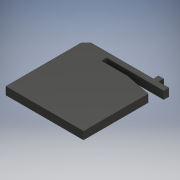
# Autodesk Inventor part: TA11
Saved by Autodesk Inventor 2017 (Build 210142000, 142)
## iProperties
Created: 2019-05-02
Part Number: TA11
Material: ABS Plastic
Document SubType Name: Modeling
Designer: Dell
Density: 1.06 g/cm^3
Appearance: Smooth - Black
Author: Dell
Autodesk Inventor part; units mm, degrees
ref_plane "YZ Plane" through (0, 0, 0) normal (1, 0, 0) x (0, 1, 0)
ref_plane "XZ Plane" through (0, 0, 0) normal (0, 1, 0) x (-1, 0, 0)
ref_plane "XY Plane" through (0, 0, 0) normal (0, 0, 1) x (1, 0, 0)
sketch "Sketch1" plane through (0, 0, 0) normal (0, 0, 1) x (1, 0, 0)
  line L0 (0, 0) -> (30, 0)
  line L1 (30, 0) -> (30, 27)
  line L2 (30, 27) -> (0, 27)
  line L3 (0, 27) -> (0, 0)
  dimension "d0" = 30
  dimension "d1" = 27
  constraints: 8 end point, 2 parallel, 1 horizontal, 1 perpendicular
  measures "d0" distance of L2.end L1.end
  measures "d1" distance of L1.end L0.end
extrude "Extrusion1" add sketch "Sketch1" along normal blind 3
sketch "Sketch2" plane through (0, 27, 0) normal (0, 1, 0) x (1, 0, 0)
  line L0 (0, 0) -> (0, -3) projected
  line L1 (0, 0) -> (30, 0) projected
  line L2 (0, -3) -> (10, -3)
  line L3 (10, -3) -> (10, 0)
  line L4 (10, 0) -> (0, 0)
  line L5 (0, 0) -> (0, -3)
  dimension "d4" = 10
  constraints: 8 end point, 2 parallel, 1 horizontal, 1 perpendicular, 1 point on line
  measures "d4" distance between parallel lines of L0 L3
extrude "Extrusion2" add sketch "Sketch2" along normal blind 2
sketch "Sketch3" plane through (0, 29, 0) normal (0, 1, 0) x (1, 0, 0)
  line L0 (0, 0) -> (0, -3) projected
  line L1 (0, -3) -> (32, -3)
  line L2 (32, -3) -> (32, 0)
  line L3 (32, 0) -> (0, 0)
  line L4 (0, 0) -> (0, -3)
  point P0 (30, 0)
  dimension "d7" = 2
  constraints: 8 end point, 2 parallel, 1 horizontal, 1 perpendicular, 1 point on line
  measures "d7" distance from line of point (30, 0) L2
extrude "Extrusion3" add sketch "Sketch3" along normal blind 2
chamfer "Chamfer1" distance 2 angle 45 1 edges at (0, 31, 1.5)
sketch "Sketch4" plane through (0, 0, 3) normal (0, 0, 1) x (1, 0, 0)
  line L0 (32, 29) -> (10, 29) projected
  line L1 (10, 29) -> (30, 25)
  line L2 (30, 0) -> (30, 27) projected
  line L3 (30, 25) -> (30, 27)
  line L4 (10, 27) -> (10, 29) projected
  line L5 (30, 27) -> (10, 29)
  line L6 (30, 0) -> (30, 27) projected
  point P0 (0, 0)
  dimension "d13" = 2
  constraints: 6 end point, 1 point on line
  measures "d13" distance of L2.end L1.end
extrude "Extrusion4" cut sketch "Sketch4" against normal through all
sketch "Sketch5" plane through (0, 0, 3) normal (0, 0, 1) x (1, 0, 0)
  line L0 (2, 31) -> (32, 31) projected
  line L1 (26, 31) -> (28, 31)
  line L2 (28, 31) -> (28, 33)
  line L3 (28, 33) -> (26, 33)
  line L4 (26, 33) -> (26, 31)
  line L5 (30, 0) -> (30, 25) projected
  point P0 (0, 0)
  dimension "d16" = 2
  dimension "d17" = 2
  dimension "d18" = 2
  constraints: 8 end point, 2 parallel, 1 horizontal, 1 perpendicular, 1 point on line
  measures "d16" distance of L3.end L2.end
  measures "d17" distance of L3.end L1.start
  measures "d18" distance between parallel lines of L2 L5
extrude "Extrusion5" add sketch "Sketch5" against normal blind 3
body "Solid1"
